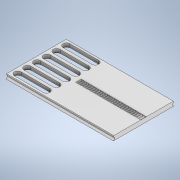
# Autodesk Inventor part: Puerta Cremallera_V2
Saved by Autodesk Inventor 2022 (Build 260153000, 153)
## iProperties
Created: 2021-02-23
Part Number: Puerta Cremallera_V2
Material: PET Plastic
Document SubType Name: Modeling
Designer: juanp
Density: 1.541 g/cm^3
Appearance: Polycarbonate - Clear
Mass: 19.6024 g
Surface Area: 162.328 cm^2
Volume: 19.6024 cm^3
Author: juanp
Autodesk Inventor part; units mm, degrees
ref_plane "YZ Plane" through (0, 0, 0) normal (1, 0, 0) x (0, 1, 0)
ref_plane "XZ Plane" through (0, 0, 0) normal (0, 1, 0) x (-1, 0, 0)
sketch "Sketch1" plane through (0, 0, 0) normal (0, 0, 1) x (1, 0, 0)
  spline S0 degree 3 poles (-1.1768, 20.967) (-1.128, 20.8639) (-1.0547, 20.7094) (-0.9668, 20.4989) (-0.9045, 20.3396) (-0.8467, 20.1786) (-0.7937, 20.0159) (-0.746, 19.8516) (-0.705, 19.6856) (-0.6701, 19.518) (-0.6556, 19.3761) (-0.6413, 19.263) (-0.626, 19.1788) (-0.6032, 19.0962) (-0.573, 19.0161) (-0.5327, 18.9404) (-0.4886, 18.8839) (-0.4476, 18.8443) (-0.4136, 18.8183) (-0.3775, 18.7952) (-0.3386, 18.7771) (-0.2983, 18.7628) (-0.2425, 18.75) (-0.1423, 18.7482) (0, 18.7512) (0.1423, 18.7482) (0.2425, 18.75) (0.2983, 18.7628) (0.3386, 18.7771) (0.3775, 18.7952) (0.4136, 18.8183) (0.4476, 18.8443) (0.4886, 18.8839) (0.5327, 18.9404) (0.573, 19.0161) (0.6032, 19.0962) (0.626, 19.1788) (0.6413, 19.263) (0.6556, 19.3761) (0.6701, 19.518) (0.705, 19.6856) (0.746, 19.8516) (0.7937, 20.0159) (0.8467, 20.1786) (0.9045, 20.3396) (0.9668, 20.4989) (1.0547, 20.7094) (1.128, 20.8639) (1.1768, 20.967) knots 0 0 0 0 0.034206 0.05131 0.068414 0.085518 0.102622 0.119726 0.136829 0.153931 0.17103 0.179582 0.188133 0.196683 0.20523 0.213776 0.222318 0.226595 0.230868 0.235144 0.239418 0.243694 0.247969 0.256512 0.273616 0.29072 0.299263 0.303538 0.307814 0.312088 0.316363 0.320637 0.324913 0.333456 0.342002 0.350549 0.359099 0.36765 0.376201 0.393301 0.410403 0.427506 0.44461 0.461714 0.478818 0.495922 0.513026 0.547232 0.547232 0.547232 0.547232
  circle A0 centre (0, 0) radius 18.75 construction
  circle A1 centre (0, 0) radius 19.363 construction
  circle A2 centre (0, 0) radius 20 construction
  circle A3 centre (0, 0) radius 21 construction
  line L0 (-1.1768, 20.967) -> (1.1768, 20.967)
  line L1 (-36.9816, 20) -> (66.9798, 20) construction
  point P0 (-1.0336, 20.6564)
  point P1 (-0.9674, 20.4986)
  point P2 (-0.9053, 20.3393)
  point P3 (-0.8475, 20.1783)
  point P4 (-0.7946, 20.0157)
  point P5 (-0.7471, 19.8514)
  point P6 (-0.706, 19.6853)
  point P7 (-0.673, 19.5175)
  point P8 (-0.6518, 19.3478)
  point P9 (-0.6405, 19.2631)
  point P10 (-0.6247, 19.179)
  point P11 (-0.602, 19.0966)
  point P12 (-0.5713, 19.0168)
  point P13 (-0.5306, 18.9417)
  point P14 (-0.4779, 18.8745)
  point P15 (-0.447, 18.8449)
  point P16 (-0.4132, 18.8187)
  point P17 (-0.377, 18.796)
  point P18 (-0.3384, 18.7778)
  point P19 (-0.298, 18.7636)
  point P20 (-0.2563, 18.7542)
  point P21 (-0.171, 18.7491)
  point P22 (0, 18.75)
  point P23 (0.171, 18.7491)
  point P24 (0.2563, 18.7542)
  point P25 (0.298, 18.7636)
  point P26 (0.3384, 18.7778)
  point P27 (0.377, 18.796)
  point P28 (0.4132, 18.8187)
  point P29 (0.447, 18.8449)
  point P30 (0.4779, 18.8745)
  point P31 (0.5306, 18.9417)
  point P32 (0.5713, 19.0168)
  point P33 (0.602, 19.0966)
  point P34 (0.6247, 19.179)
  point P35 (0.6405, 19.2631)
  point P36 (0.6518, 19.3478)
  point P37 (0.673, 19.5175)
  point P38 (0.706, 19.6853)
  point P39 (0.7471, 19.8514)
  point P40 (0.7946, 20.0157)
  point P41 (0.8475, 20.1783)
  point P42 (0.9053, 20.3393)
  point P43 (0.9674, 20.4986)
  point P44 (1.0336, 20.6564)
  constraints: 4 centre point, 4 end point, 2 horizontal, 2 point on circle, 1 tangent, 99 other
sketch "Sketch2" plane through (0, 0, 0) normal (0, 0, 1) x (1, 0, 0)
  line L0 (-3.6768, 20.967) -> (86.3232, 20.967)
  line L1 (86.3232, 20.967) -> (86.3232, 17.967)
  line L2 (86.3232, 17.967) -> (-3.6768, 17.967)
  line L3 (-3.6768, 17.967) -> (-3.6768, 20.967)
  point P0 (0, 0)
  point P1 (-1.1768, 20.967)
  point P2 (1.1768, 20.967)
  dimension "d2" = 3
  dimension "d3" = 2.5
  dimension "d4" = 90
  constraints: 8 end point, 2 parallel, 1 horizontal, 1 perpendicular, 1 point on line
  measures "d2" distance between parallel lines of L0 L2
  measures "d3" distance of L0.start point (-1.177, 20.967)
  measures "d4" distance between parallel lines of L3 L1
extrude "Extrusion2" add sketch "Sketch2" along normal mid plane 80.1
extrude "Extrusion3" cut sketch "Sketch1" along normal mid plane 7.5
pattern_linear "Rectangular Pattern1" count 28 spacing 3.1416 along (1, 0, 0) of "Extrusion3"
ref_plane "Work Plane1" through (-36.9816, 20, 0) normal (0, 1, 0) x (1, 0, 0)
sketch "Sketch4" plane through (-3.6768, 20.967, 40.05) normal (0, 1, 0) x (1, 0, 0)
  line L0 (-57.967, 187.7557) -> (-57.967, 106.7557) construction
  line L1 (-3.967, 176.4057) -> (-3.967, 187.7557) construction
  line L2 (-3.967, 106.7557) -> (-3.967, 151.4057) construction
  line L3 (-50.3837, 185.7557) -> (-11.5504, 185.7557) construction
  line L4 (-11.5504, 185.7557) -> (-50.3837, 185.7557) construction
  line L5 (-50.3837, 172.589) -> (-11.5504, 172.589) construction
  line L6 (-11.5504, 172.589) -> (-50.3837, 172.589) construction
  line L7 (-50.3837, 159.4224) -> (-11.5504, 159.4224) construction
  line L8 (-11.5504, 159.4224) -> (-50.3837, 159.4224) construction
  line L9 (-50.3837, 146.2557) -> (-11.5504, 146.2557) construction
  line L10 (-11.5504, 146.2557) -> (-50.3837, 146.2557) construction
  line L11 (-50.3837, 133.089) -> (-11.5504, 133.089) construction
  line L12 (-11.5504, 133.089) -> (-50.3837, 133.089) construction
  line L13 (-50.3837, 119.9224) -> (-11.5504, 119.9224) construction
  line L14 (-11.5504, 119.9224) -> (-50.3837, 119.9224) construction
  arc A0 (-50.3837, 119.9224) -> (-50.3837, 108.7557) centre (-50.3837, 114.339) ccw construction
  arc A1 (-55.967, 114.339) -> (-50.3837, 108.7557) centre (-50.3837, 114.339) ccw construction
  arc A2 (-50.3837, 119.9224) -> (-55.967, 114.339) centre (-50.3837, 114.339) ccw construction
  arc A3 (-50.3837, 133.089) -> (-50.3837, 121.9224) centre (-50.3837, 127.5057) ccw construction
  arc A4 (-55.967, 127.5057) -> (-50.3837, 121.9224) centre (-50.3837, 127.5057) ccw construction
  arc A5 (-50.3837, 133.089) -> (-55.967, 127.5057) centre (-50.3837, 127.5057) ccw construction
  arc A6 (-50.3837, 146.2557) -> (-50.3837, 135.089) centre (-50.3837, 140.6724) ccw construction
  arc A7 (-55.967, 140.6724) -> (-50.3837, 135.089) centre (-50.3837, 140.6724) ccw construction
  arc A8 (-50.3837, 146.2557) -> (-55.967, 140.6724) centre (-50.3837, 140.6724) ccw construction
  arc A9 (-50.3837, 159.4224) -> (-50.3837, 148.2557) centre (-50.3837, 153.839) ccw construction
  arc A10 (-55.967, 153.839) -> (-50.3837, 148.2557) centre (-50.3837, 153.839) ccw construction
  arc A11 (-50.3837, 159.4224) -> (-55.967, 153.839) centre (-50.3837, 153.839) ccw construction
  arc A12 (-50.3837, 172.589) -> (-50.3837, 161.4224) centre (-50.3837, 167.0057) ccw construction
  arc A13 (-55.967, 167.0057) -> (-50.3837, 161.4224) centre (-50.3837, 167.0057) ccw construction
  arc A14 (-50.3837, 172.589) -> (-55.967, 167.0057) centre (-50.3837, 167.0057) ccw construction
  arc A15 (-50.3837, 185.7557) -> (-50.3837, 174.589) centre (-50.3837, 180.1724) ccw construction
  arc A16 (-55.967, 180.1724) -> (-50.3837, 174.589) centre (-50.3837, 180.1724) ccw construction
  arc A17 (-50.3837, 185.7557) -> (-55.967, 180.1724) centre (-50.3837, 180.1724) ccw construction
  arc A18 (-11.5504, 174.589) -> (-11.5504, 185.7557) centre (-11.5504, 180.1724) ccw construction
  arc A19 (-5.967, 180.1724) -> (-11.5504, 185.7557) centre (-11.5504, 180.1724) ccw construction
  arc A20 (-11.5504, 174.589) -> (-5.967, 180.1724) centre (-11.5504, 180.1724) ccw construction
  arc A21 (-11.5504, 161.4224) -> (-11.5504, 172.589) centre (-11.5504, 167.0057) ccw construction
  arc A22 (-5.967, 167.0057) -> (-11.5504, 172.589) centre (-11.5504, 167.0057) ccw construction
  arc A23 (-11.5504, 161.4224) -> (-5.967, 167.0057) centre (-11.5504, 167.0057) ccw construction
  arc A24 (-11.5504, 148.2557) -> (-11.5504, 159.4224) centre (-11.5504, 153.839) ccw construction
  arc A25 (-5.967, 153.839) -> (-11.5504, 159.4224) centre (-11.5504, 153.839) ccw construction
  arc A26 (-11.5504, 148.2557) -> (-5.967, 153.839) centre (-11.5504, 153.839) ccw construction
  arc A27 (-11.5504, 135.089) -> (-11.5504, 146.2557) centre (-11.5504, 140.6724) ccw construction
  arc A28 (-5.967, 140.6724) -> (-11.5504, 146.2557) centre (-11.5504, 140.6724) ccw construction
  arc A29 (-11.5504, 135.089) -> (-5.967, 140.6724) centre (-11.5504, 140.6724) ccw construction
  arc A30 (-11.5504, 121.9224) -> (-11.5504, 133.089) centre (-11.5504, 127.5057) ccw construction
  arc A31 (-5.967, 127.5057) -> (-11.5504, 133.089) centre (-11.5504, 127.5057) ccw construction
  arc A32 (-11.5504, 121.9224) -> (-5.967, 127.5057) centre (-11.5504, 127.5057) ccw construction
  arc A33 (-11.5504, 108.7557) -> (-11.5504, 119.9224) centre (-11.5504, 114.339) ccw construction
  arc A34 (-5.967, 114.339) -> (-11.5504, 119.9224) centre (-11.5504, 114.339) ccw construction
  arc A35 (-11.5504, 108.7557) -> (-5.967, 114.339) centre (-11.5504, 114.339) ccw construction
  line L15 (-11.5504, 108.7557) -> (-50.3837, 108.7557) construction
  line L16 (-50.3837, 108.7557) -> (-11.5504, 108.7557) construction
  line L17 (-11.5504, 121.9224) -> (-50.3837, 121.9224) construction
  line L18 (-50.3837, 121.9224) -> (-11.5504, 121.9224) construction
  line L19 (-11.5504, 135.089) -> (-50.3837, 135.089) construction
  line L20 (-50.3837, 135.089) -> (-11.5504, 135.089) construction
  line L21 (-11.5504, 148.2557) -> (-50.3837, 148.2557) construction
  line L22 (-50.3837, 148.2557) -> (-11.5504, 148.2557) construction
  line L23 (-11.5504, 161.4224) -> (-50.3837, 161.4224) construction
  line L24 (-50.3837, 161.4224) -> (-11.5504, 161.4224) construction
  line L25 (-11.5504, 174.589) -> (-50.3837, 174.589) construction
  line L26 (-50.3837, 174.589) -> (-11.5504, 174.589) construction
  line L27 (-57.967, 106.7557) -> (-3.967, 106.7557) construction
  line L28 (-3.967, 187.7557) -> (-57.967, 187.7557) construction
  line L29 (0, 80.1) -> (0, 0) projected
  line L30 (0, 0) -> (-54, 0)
  line L31 (-54, 0) -> (-54, 80.1)
  line L32 (-54, 80.1) -> (0, 80.1)
  line L33 (-7.5835, 1.8) -> (-46.4165, 1.8)
  arc A36 (-46.4165, 12.8833) -> (-46.4165, 1.8) centre (-46.4165, 7.3417) ccw
  line L34 (-46.4165, 12.8833) -> (-7.5835, 12.8833)
  arc A37 (-7.5835, 1.8) -> (-7.5835, 12.8833) centre (-7.5835, 7.3417) ccw
  arc A38 (-46.4165, 25.9667) -> (-46.4165, 14.8833) centre (-46.4165, 20.425) ccw
  line L35 (-7.5835, 14.8833) -> (-46.4165, 14.8833)
  line L36 (-46.4165, 25.9667) -> (-7.5835, 25.9667)
  arc A39 (-7.5835, 14.8833) -> (-7.5835, 25.9667) centre (-7.5835, 20.425) ccw
  arc A40 (-46.4165, 39.05) -> (-46.4165, 27.9667) centre (-46.4165, 33.5083) ccw
  line L37 (-7.5835, 27.9667) -> (-46.4165, 27.9667)
  line L38 (-46.4165, 39.05) -> (-7.5835, 39.05)
  arc A41 (-7.5835, 27.9667) -> (-7.5835, 39.05) centre (-7.5835, 33.5083) ccw
  arc A42 (-46.4165, 52.1333) -> (-46.4165, 41.05) centre (-46.4165, 46.5917) ccw
  line L39 (-7.5835, 41.05) -> (-46.4165, 41.05)
  line L40 (-46.4165, 52.1333) -> (-7.5835, 52.1333)
  arc A43 (-7.5835, 41.05) -> (-7.5835, 52.1333) centre (-7.5835, 46.5917) ccw
  arc A44 (-46.4165, 65.2167) -> (-46.4165, 54.1333) centre (-46.4165, 59.675) ccw
  line L41 (-7.5835, 54.1333) -> (-46.4165, 54.1333)
  line L42 (-46.4165, 65.2167) -> (-7.5835, 65.2167)
  arc A45 (-7.5835, 54.1333) -> (-7.5835, 65.2167) centre (-7.5835, 59.675) ccw
  arc A46 (-46.4165, 78.3) -> (-46.4165, 67.2167) centre (-46.4165, 72.7583) ccw
  line L43 (-7.5835, 67.2167) -> (-46.4165, 67.2167)
  line L44 (-46.4165, 78.3) -> (-7.5835, 78.3)
  arc A47 (-7.5835, 67.2167) -> (-7.5835, 78.3) centre (-7.5835, 72.7583) ccw
  line L45 (-27, 78.3) -> (-27, 80.1) construction
  line L46 (-27, 1.8) -> (-27, 0) construction
  line L47 (-7.5835, 11.8833) -> (-46.4165, 11.8833)
  arc A48 (-46.4165, 11.8833) -> (-46.4165, 2.8) centre (-46.4165, 7.3417) ccw
  line L48 (-46.4165, 2.8) -> (-7.5835, 2.8)
  arc A49 (-7.5835, 2.8) -> (-7.5835, 11.8833) centre (-7.5835, 7.3417) ccw
  arc A50 (-7.5835, 15.8833) -> (-7.5835, 24.9667) centre (-7.5835, 20.425) ccw
  line L49 (-7.5835, 24.9667) -> (-46.4165, 24.9667)
  line L50 (-46.4165, 15.8833) -> (-7.5835, 15.8833)
  arc A51 (-46.4165, 24.9667) -> (-46.4165, 15.8833) centre (-46.4165, 20.425) ccw
  arc A52 (-7.5835, 28.9667) -> (-7.5835, 38.05) centre (-7.5835, 33.5083) ccw
  line L51 (-7.5835, 38.05) -> (-46.4165, 38.05)
  line L52 (-46.4165, 28.9667) -> (-7.5835, 28.9667)
  arc A53 (-46.4165, 38.05) -> (-46.4165, 28.9667) centre (-46.4165, 33.5083) ccw
  arc A54 (-7.5835, 42.05) -> (-7.5835, 51.1333) centre (-7.5835, 46.5917) ccw
  line L53 (-7.5835, 51.1333) -> (-46.4165, 51.1333)
  line L54 (-46.4165, 42.05) -> (-7.5835, 42.05)
  arc A55 (-46.4165, 51.1333) -> (-46.4165, 42.05) centre (-46.4165, 46.5917) ccw
  arc A56 (-7.5835, 55.1333) -> (-7.5835, 64.2167) centre (-7.5835, 59.675) ccw
  line L55 (-7.5835, 64.2167) -> (-46.4165, 64.2167)
  line L56 (-46.4165, 55.1333) -> (-7.5835, 55.1333)
  arc A57 (-46.4165, 64.2167) -> (-46.4165, 55.1333) centre (-46.4165, 59.675) ccw
  arc A58 (-7.5835, 68.2167) -> (-7.5835, 77.3) centre (-7.5835, 72.7583) ccw
  line L57 (-7.5835, 77.3) -> (-46.4165, 77.3)
  line L58 (-46.4165, 68.2167) -> (-7.5835, 68.2167)
  arc A59 (-46.4165, 77.3) -> (-46.4165, 68.2167) centre (-46.4165, 72.7583) ccw
  point P0 (3.6768, 40.05)
  dimension "d22" = 54
  dimension "d23" = 5.5417
  dimension "d24" = 38.833
  dimension "d27" = 13.0833
  dimension "d38" = 1
  dimension "d41" = 13.0833
  constraints: 120 point on circle, 116 end point, 60 centre point, 4 midpoint, 4 perpendicular, 3 horizontal, 3 tangent, 2 vertical, 1 collinear, 1 equal radius, 103 other
  measures "d22" distance of L31.end L29.start
  measures "d23" radius of A36
  measures "d24" distance of L34.start L34.end
  measures "d27" distance of A36.centre A38.centre
  measures "d38" distance between parallel lines of L48 L33
  measures "d41" distance of A37.centre A50.centre
extrude "Extrusion5" add sketch "Sketch4" against normal up to surface (3 mm away) contours L29 L30 L31 L32 | L33 A36 L34 A37 | L36 A39 L35 A38 | L38 A41 L37 A40 | L40 A43 L39 A42 | L42 A45 L41 A44 | L44 A47 L43 A46
chamfer "Chamfer1" distance 1.416 angle 45 2 edges at (14.3232, 17.967, 40.05) (14.3232, 17.967, -40.05)
sketch "Sketch7" plane through (-57.6768, 17.967, -38.634) normal (0, -1, 0) x (1, 0, 0)
  line L0 (144, 0) -> (0, 0) projected
  line L1 (144, 0) -> (144, 77.268) projected
  line L2 (0, 77.268) -> (144, 77.268) projected
  line L3 (0, 0) -> (0, 77.268) projected
  arc A0 (7.5835, 10.4673) -> (7.5835, 1.384) centre (7.5835, 5.9257) ccw projected
  line L4 (46.4165, 10.4673) -> (7.5835, 10.4673) projected
  arc A1 (46.4165, 1.384) -> (46.4165, 10.4673) centre (46.4165, 5.9257) ccw projected
  line L5 (7.5835, 1.384) -> (46.4165, 1.384) projected
  arc A2 (7.5835, 23.5507) -> (7.5835, 14.4673) centre (7.5835, 19.009) ccw projected
  line L6 (46.4165, 23.5507) -> (7.5835, 23.5507) projected
  arc A3 (46.4165, 14.4673) -> (46.4165, 23.5507) centre (46.4165, 19.009) ccw projected
  line L7 (7.5835, 14.4673) -> (46.4165, 14.4673) projected
  arc A4 (7.5835, 36.634) -> (7.5835, 27.5507) centre (7.5835, 32.0923) ccw projected
  line L8 (46.4165, 36.634) -> (7.5835, 36.634) projected
  arc A5 (46.4165, 27.5507) -> (46.4165, 36.634) centre (46.4165, 32.0923) ccw projected
  line L9 (7.5835, 27.5507) -> (46.4165, 27.5507) projected
  arc A6 (7.5835, 49.7173) -> (7.5835, 40.634) centre (7.5835, 45.1757) ccw projected
  line L10 (46.4165, 49.7173) -> (7.5835, 49.7173) projected
  arc A7 (46.4165, 40.634) -> (46.4165, 49.7173) centre (46.4165, 45.1757) ccw projected
  line L11 (7.5835, 40.634) -> (46.4165, 40.634) projected
  arc A8 (7.5835, 62.8007) -> (7.5835, 53.7173) centre (7.5835, 58.259) ccw projected
  line L12 (46.4165, 62.8007) -> (7.5835, 62.8007) projected
  arc A9 (46.4165, 53.7173) -> (46.4165, 62.8007) centre (46.4165, 58.259) ccw projected
  line L13 (7.5835, 53.7173) -> (46.4165, 53.7173) projected
  line L14 (46.4165, 75.884) -> (7.5835, 75.884) projected
  arc A10 (46.4165, 66.8007) -> (46.4165, 75.884) centre (46.4165, 71.3423) ccw projected
  line L15 (7.5835, 66.8007) -> (46.4165, 66.8007) projected
  arc A11 (7.5835, 75.884) -> (7.5835, 66.8007) centre (7.5835, 71.3423) ccw projected
  point P0 (57.6768, 38.634)
extrude "Extrusion7" add sketch "Sketch7" along normal blind 1
sketch "Sketch8" plane through (-57.6768, 16.967, -38.634) normal (0, -1, 0) x (1, 0, 0)
  line L0 (0, -1.416) -> (0, 78.684) projected
  line L1 (0, 77.268) -> (144, 77.268) projected
  line L2 (0, 75.884) -> (144, 75.884)
  line L3 (144, 75.884) -> (144, 77.268)
  line L4 (144, 77.268) -> (0, 77.268)
  line L5 (0, 77.268) -> (0, 75.884)
  line L6 (7.5835, 75.884) -> (46.4165, 75.884) projected
  point P0 (57.6768, 38.634)
  constraints: 8 end point, 2 parallel, 1 collinear, 1 horizontal, 1 perpendicular, 1 point on line
sketch "Sketch9" plane through (86.3232, 20.967, 40.05) normal (1, 0, 0) x (0, 0, -1)
  line L0 (1.416, -3) -> (1.416, -4) projected
  line L1 (1.416, -4) -> (-0.584, -6)
  line L2 (78.684, -4) -> (1.416, -4) projected
  point P0 (40.05, -20.967)
  dimension "d46" = 45
  dimension "d49" = 2
  constraints: 2 end point
  measures "d46" angle of L1 L2
  measures "d49" distance from line of L1.end L2
sweep "Sweep1" add profiles "Sketch8" path "Sketch9" path curves L1
mirror "Mirror1" about plane through (0, 0, 0) normal (0, 0, 1) of "Sweep1"
sketch "Sketch10" plane through (-57.6768, 14.967, -40.634) normal (0, -1, 0) x (1, 0, 0)
  line L0 (46.4165, 3.384) -> (144, 3.384) projected
  line L1 (144, 3.384) -> (144, 77.884) projected
  line L2 (144, 77.884) -> (46.4165, 77.884) construction
  arc A0 (46.4165, 68.8007) -> (46.4165, 77.884) centre (46.4165, 73.3423) ccw projected
  line L3 (46.4165, 68.8007) -> (7.5835, 68.8007) projected
  arc A1 (7.5835, 77.884) -> (7.5835, 68.8007) centre (7.5835, 73.3423) ccw projected
  line L4 (7.5835, 77.884) -> (0, 77.884) projected
  line L5 (0, 77.884) -> (0, 3.384) projected
  line L6 (0, 3.384) -> (7.5835, 3.384) projected
  arc A2 (7.5835, 12.4673) -> (7.5835, 3.384) centre (7.5835, 7.9257) ccw projected
  line L7 (7.5835, 12.4673) -> (46.4165, 12.4673) projected
  arc A3 (46.4165, 3.384) -> (46.4165, 12.4673) centre (46.4165, 7.9257) ccw projected
  line L8 (7.5835, 25.5507) -> (46.4165, 25.5507) projected
  arc A4 (46.4165, 16.4673) -> (46.4165, 25.5507) centre (46.4165, 21.009) ccw projected
  line L9 (46.4165, 16.4673) -> (7.5835, 16.4673) projected
  arc A5 (7.5835, 25.5507) -> (7.5835, 16.4673) centre (7.5835, 21.009) ccw projected
  line L10 (7.5835, 38.634) -> (46.4165, 38.634) projected
  arc A6 (46.4165, 29.5507) -> (46.4165, 38.634) centre (46.4165, 34.0923) ccw projected
  line L11 (46.4165, 29.5507) -> (7.5835, 29.5507) projected
  arc A7 (7.5835, 38.634) -> (7.5835, 29.5507) centre (7.5835, 34.0923) ccw projected
  line L12 (7.5835, 51.7173) -> (46.4165, 51.7173) projected
  arc A8 (46.4165, 42.634) -> (46.4165, 51.7173) centre (46.4165, 47.1757) ccw projected
  line L13 (46.4165, 42.634) -> (7.5835, 42.634) projected
  arc A9 (7.5835, 51.7173) -> (7.5835, 42.634) centre (7.5835, 47.1757) ccw projected
  line L14 (7.5835, 64.8007) -> (46.4165, 64.8007) projected
  arc A10 (46.4165, 55.7173) -> (46.4165, 64.8007) centre (46.4165, 60.259) ccw projected
  line L15 (46.4165, 55.7173) -> (7.5835, 55.7173) projected
  arc A11 (7.5835, 64.8007) -> (7.5835, 55.7173) centre (7.5835, 60.259) ccw projected
  line L16 (0, 3.384) -> (7.5835, 3.384) projected
  line L17 (0, 3.384) -> (0, 1.384) projected
  line L18 (0, 1.384) -> (144, 1.384) projected
  line L19 (144, 3.384) -> (144, 1.384) projected
  line L20 (46.4165, 3.384) -> (144, 3.384) construction
  line L21 (46.4165, 3.384) -> (7.5835, 3.384) projected
  line L22 (7.5835, 77.884) -> (0, 77.884) projected
  line L23 (7.5835, 77.884) -> (46.4165, 77.884) projected
  line L24 (144, 77.884) -> (46.4165, 77.884) projected
  line L25 (144, 77.884) -> (144, 79.884) projected
  line L26 (0, 79.884) -> (144, 79.884) projected
  line L27 (0, 77.884) -> (0, 79.884) projected
  point P0 (57.6768, 40.634)
  point P1 (0, 3.384)
  point P2 (46.4165, 77.884)
  point P3 (7.5835, 77.884)
  point P4 (46.4165, 3.384)
  point P5 (7.5835, 3.384)
extrude "Extrusion8" add sketch "Sketch10" against normal up to next contours A3 L7 A2 L6 L5 L4 A1 L3 A0 L24 L1 L0 | L0 L19 L18 L17 L6 L21 | L24 L23 L4 L27 L26 L25
chamfer "Chamfer8" distance 1.5 angle 45 24 edges at (-6.7186, 14.967, 32.7083) (-30.6768, 14.967, 28.1667) (-54.635, 14.967, 32.7083) (-30.6768, 14.967, 37.25) (-6.7186, 14.967, 19.625) (-30.6768, 14.967, 15.0833) (-54.635, 14.967, 19.625) (-30.6768, 14.967, 24.1667) (-6.7186, 14.967, 6.5417) (-30.6768, 14.967, 2) (-54.635, 14.967, 6.5417) (-30.6768, 14.967, 11.0833) (-6.7186, 14.967, -19.625) (-30.6768, 14.967, -24.1667) (-54.635, 14.967, -19.625) (-30.6768, 14.967, -15.0833) (-6.7186, 14.967, -32.7083) (-30.6768, 14.967, -37.25) (-54.635, 14.967, -32.7083) (-30.6768, 14.967, -28.1667) (-6.7186, 14.967, -6.5417) (-30.6768, 14.967, -11.0833) (-54.635, 14.967, -6.5417) (-30.6768, 14.967, -2)
equation "\"Module\" = 1"
equation "\"PressureAngle\" = 14.5deg"
equation "\"UnitProfileClearance\" = 0.25"
equation "\"UnitRoundRadius\" = 0.3335"
equation "\"HeadDiameter\" = 42"
equation "\"RootDiameter\" = 37.5"
equation "\"BaseDiameter\" = 38.72591"
equation "\"FaceWidth\" = 5"
equation "\"HelixAngle\" = 0"
equation "\"UnitCorrection\" = 0"
equation "\"UnitAddendumModification\" = 0"
equation "\"CircularPitch\" = 3.141593"
equation "\"UnitBacklashShift\" = 0"
equation "\"TotalToolShift\" = 0"
equation "\"IsInternal\" = 0"
body "Solid2"
